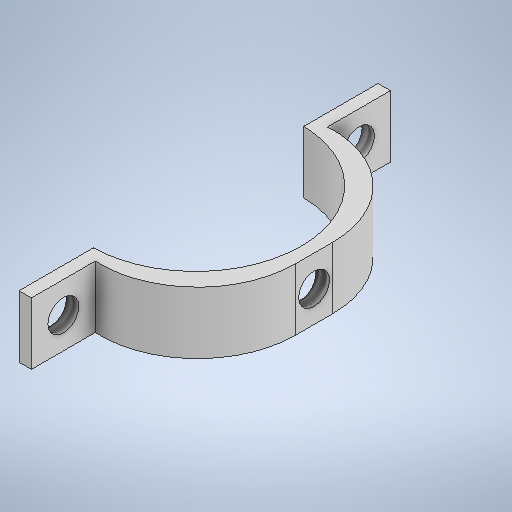
# Autodesk Inventor part: obejma_fi32_L44
Saved by Autodesk Inventor 2025.2 (Build 292293000, 293)
## iProperties
Created: 2025-03-20
Part Number: obejma_fi32_L44
Material: Ogólny
Document SubType Name: Modeling
Designer: rango
Density: 1 g/cm^3
Appearance: Domyślna
Author: rango
Autodesk Inventor part; units mm, degrees
ref_plane "YZ Plane" through (0, 0, 0) normal (1, 0, 0) x (0, 1, 0)
ref_plane "XZ Plane" through (0, 0, 0) normal (0, 1, 0) x (-1, 0, 0)
sketch "Szkic1" plane through (0, 0, 0) normal (0, 1, 0) x (-1, 0, 0)
  line L0 (0, 17) -> (0, -17) construction
  line L1 (0, 0) -> (-17, 0)
  line L2 (0, 17) -> (0, 19)
  line L3 (0, -17) -> (0, -19)
  line L4 (-16.5569, 0) -> (-18.5569, 0)
  line L5 (0, 19) -> (0, 29)
  line L6 (0, 29) -> (-2, 29)
  line L7 (-2, 29) -> (-2, 18.7083)
  line L8 (0, -19) -> (0, -29)
  line L9 (0, -29) -> (-2, -29)
  line L10 (-2, -29) -> (-2, -18.8469)
  line L11 (-18.5573, 2.8889) -> (-18.5573, -3.1111)
  arc A0 (-2, 18.7083) -> (-18.5573, 2.8889) centre (-2.7215, 2.8889) ccw
  arc A1 (-18.5573, -3.1111) -> (-2, -18.8469) centre (-2.8011, -3.1111) ccw
  arc A2 (0, 17) -> (0, -17) centre (0.449, 0) ccw
  dimension "d0" = 34
  dimension "d1" = 17
  dimension "d2" = 2
  dimension "d3" = 2
  dimension "d4" = 2
  dimension "d5" = 10
  dimension "d6" = 2
  dimension "d7" = 10
  dimension "d8" = 2
  dimension "d41" = 6
  constraints: 24 end point, 7 point on circle, 5 vertical, 3 centre point, 3 point on line, 2 horizontal, 2 perpendicular, 2 tangent
  measures "d0" distance of L0.start L0.end
  measures "d1" distance of L1.start L1.end
  measures "d2" distance of L0.start L2.end
  measures "d3" distance of L0.end L3.end
  measures "d4" distance of L4.start L4.end
  measures "d5" distance of L2.end L5.end
  measures "d6" distance of L5.end L6.end
  measures "d7" distance of L3.end L8.end
  measures "d8" distance of L8.end L9.end
  measures "d41" distance of L11.start L11.end
ref_plane "Płaszczyzna konstrukcyjna1" through (0, 0, 17) normal (-1, 0, 0) x (0, 0, 1)
extrude "Wyciągnięcie proste3" add sketch "Szkic1" along normal blind 10
sketch "Szkic4" plane through (0, 0, -29) normal (-1, 0, 0) x (0, 0, 1)
  line L0 (10.1531, 0) -> (10.1531, 10) projected
  line L1 (10.1531, 5) -> (0, 5) construction
  line L2 (0, 0) -> (0, 10) projected
  line L3 (10.1531, 10) -> (0, 10) projected
  line L4 (5.0765, 10) -> (5.0765, 0) construction
  line L5 (10.1531, 0) -> (0, 0) projected
  line L6 (47.7083, 0) -> (47.7083, 10) projected
  line L7 (47.7083, 5) -> (58, 5) construction
  line L8 (58, 0) -> (58, 10) projected
  line L9 (46, 10) -> (58, 10) projected
  line L10 (52.8541, 10) -> (52.8541, 0) construction
  circle A0 centre (52.8541, 5) radius 3
  circle A1 centre (5.0765, 5) radius 3
  point P0 (29, 0)
  dimension "d45" = 6
  dimension "d46" = 6
  constraints: 8 end point, 8 midpoint, 2 centre point, 1 perpendicular, 1 point on line
  measures "d45" diameter of A0
  measures "d46" diameter of A1
hole "Otwór4" at (0, 5, -23.9235) at (0, 5, 23.8541) direction (1, 0, 0) diameter 4.9784 depth 19.05 tip angle 118 thread size "1/4-20 UNC" class "2B" standard "ANSI Unified Screw Threads"
sketch "Szkic5" plane through (18.5573, 0, 2.8889) normal (1, 0, 0) x (0, 0, -1)
  line L0 (0, 10) -> (6, 10) projected
  line L1 (3, 10) -> (3, 0)
  line L2 (0, 0) -> (6, 0) projected
  line L3 (0, 0) -> (0, 10) projected
  line L4 (0, 5) -> (6, 5)
  line L5 (6, 0) -> (6, 10) projected
  circle A0 centre (3, 5) radius 3
  point P0 (2.8889, 0)
  dimension "d54" = 6
  constraints: 5 midpoint, 4 end point, 1 centre point
  measures "d54" diameter of A0
hole "Otwór5" at (18.5573, 5, -0.1111) direction (-1, 0, 0) diameter 4.9784 depth 19.05 tip angle 118 thread size "1/4-20 UNC" class "2B" standard "ANSI Unified Screw Threads"
